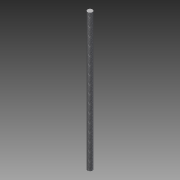
# Autodesk Inventor part: Gewindestange3
Saved by Autodesk Inventor 2013 (Build 170138000, 138)
## iProperties
Created: 2012-12-21
Part Number: Gewindestange3
Material: Stahl
Document SubType Name: Modeling
Designer: Lukas
Density: 7.85 g/cm^3
Mass: 6.65861 g
Surface Area: 11.4511 cm^2
Volume: 0.84823 cm^3
Author: Lukas
Autodesk Inventor part; units mm, degrees
ref_plane "YZ Plane" through (0, 0, 0) normal (1, 0, 0) x (0, 1, 0)
ref_plane "XZ Plane" through (0, 0, 0) normal (0, 1, 0) x (-1, 0, 0)
ref_plane "XY Plane" through (0, 0, 0) normal (0, 0, 1) x (1, 0, 0)
sketch "Skizze1" plane through (0, 0, 0) normal (0, 0, 1) x (1, 0, 0)
  circle A0 centre (0, 0) radius 2.5
  dimension "d0" = 5
  constraints: 1 centre point, 1 coincident
  measures "d0" diameter of A0
extrude "Extrusion1" add sketch "Skizze1" along normal blind 140
thread "Gewinde2" size "M5x0.8" class "6g" standard "ANSI Metric M Profile" full length
